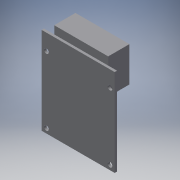
# Autodesk Inventor part: board
Saved by Autodesk Inventor 2018 (Build 220112000, 112)
## iProperties
Created: 2018-06-29
Part Number: board
Material: Generic
Document SubType Name: Modeling
Designer: erwin
Density: 1 g/cm^3
Appearance: Default
Author: erwin
Autodesk Inventor part; units mm, degrees
ref_plane "YZ Plane" through (0, 0, 0) normal (1, 0, 0) x (0, 1, 0)
ref_plane "XZ Plane" through (0, 0, 0) normal (0, 1, 0) x (-1, 0, 0)
ref_plane "XY Plane" through (0, 0, 0) normal (0, 0, 1) x (1, 0, 0)
sketch "Sketch1" plane through (0, 0, 0) normal (0, 1, 0) x (-1, 0, 0)
  line L0 (-23, 27.5) -> (23, 27.5)
  line L1 (23, 27.5) -> (23, -27.5)
  line L2 (23, -27.5) -> (-23, -27.5)
  line L3 (-23, -27.5) -> (-23, 27.5)
  line L4 (-23, 27.5) -> (23, -27.5) construction
  line L5 (23, 27.5) -> (-23, -27.5) construction
  point P0 (0, 0)
  dimension "d0" = 46
  dimension "d1" = 55
  constraints: 12 end point, 2 midpoint, 2 parallel, 1 horizontal, 1 perpendicular
  measures "d0" distance of L1.end L2.end
  measures "d1" distance of L0.end L1.end
extrude "Extrusion1" add sketch "Sketch1" along normal blind 1.5
sketch "Sketch2" plane through (0, 1.5, 0) normal (0, 1, 0) x (1, 0, 0)
  line L0 (-16.6, -32.5) -> (17.4, -32.5)
  line L1 (17.4, -32.5) -> (17.4, -10.5)
  line L2 (17.4, -10.5) -> (-16.6, -10.5)
  line L3 (-16.6, -10.5) -> (-16.6, -32.5)
  line L4 (-16.6, -32.5) -> (17.4, -10.5) construction
  line L5 (17.4, -32.5) -> (-16.6, -10.5) construction
  line L6 (-23, -27.5) -> (23, -27.5) projected
  line L7 (-23, 27.5) -> (-23, -27.5) projected
  point P0 (0, 0)
  point P1 (0.4, -21.5)
  dimension "d4" = 34
  dimension "d5" = 22
  dimension "d6" = 5
  dimension "d7" = 6.4
  constraints: 12 end point, 2 midpoint, 2 parallel, 1 horizontal, 1 perpendicular
  measures "d4" distance of L2.end L1.end
  measures "d5" distance of L1.end L0.end
  measures "d6" distance between parallel lines of L6 L0
  measures "d7" distance between parallel lines of L7 L3
extrude "Extrusion2" add sketch "Sketch2" along normal blind 13.4
sketch "Sketch3" plane through (0, 0, 0) normal (0, -1, 0) x (1, 0, 0)
  line L0 (20, 17.5) -> (-20, 17.5) construction
  line L1 (-20, 17.5) -> (-20, -24.5) construction
  line L2 (-20, -24.5) -> (20, -24.5) construction
  line L3 (20, -24.5) -> (20, 17.5) construction
  line L4 (23, -27.5) -> (23, 27.5) construction
  line L5 (-23, 27.5) -> (-23, -27.5) projected
  line L6 (-23, -27.5) -> (23, -27.5) projected
  point P0 (0, 0)
  dimension "d10" = 42
  dimension "d11" = 40
  dimension "d12" = 3
  dimension "d13" = 3
  dimension "d14" = 3
  constraints: 8 end point, 4 coincident, 2 parallel, 1 horizontal, 1 perpendicular
  measures "d10" distance of L2.end L0.start
  measures "d11" distance of L1.end L2.end
  measures "d12" distance between parallel lines of L4 L3
  measures "d13" distance between parallel lines of L5 L1
  measures "d14" distance between parallel lines of L6 L2
hole "Hole1" at (20, 0, 17.5) at (-20, 0, 17.5) at (-20, 0, -24.5) at (20, 0, -24.5) direction (0, 1, 0) diameter 3 end through all
equation "\"d13\" = d12"
equation "\"d14\" = d12"
body "Solid1"
